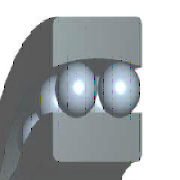
# Autodesk Inventor part: Подшипник 1212 ГОСТ 28428-90
Saved by Autodesk Inventor 2021 (Build 250183000, 183)
## iProperties
Created: 2020-01-21
Part Number: Подшипник 1212 ГОСТ 28428-90
Material: Сталь, мягкая
Description: ПОДШИПНИКИ РАДИАЛЬНЫЕ ШАРИКОВЫЕ СФЕРИЧЕСКИЕ ДВУХРЯДНЫЕ
Document SubType Name: Modeling
Standard: ГОСТ 28428-90
Designer: gdevc
Standards Organization: GOST
Language: ru-RU
Size Designation: 1212
Categories: <MemberInstance><Categories><Category DisplayName="Детали вала" InternalName="7f7aeb1f-a693-4053-b835-cee3144e0d98" Mnemonic="SHFT"><Category DisplayName="Подшипники" InternalName="242d30a3-7172-44e6-a363-b0a3d8f1b556" Mnemonic="BRNG"><CategoryParameter DisplayName="Ширина" InternalName="25fc5f6e-338b-4801-b5ed-8959743e396e" Mnemonic="wdth"/><CategoryParameter DisplayName="Обозначение размера" InternalName="2c4e891a-c8f4-49ed-a5c1-5131476c6feb" Mnemonic="sizedes"/><CategoryParameter DisplayName="Номинальная динамическая нагрузка" InternalName="440972dd-7009-4861-bd45-69ffbb461423" Mnemonic="bdynlrat"/><CategoryParameter DisplayName="Диаметр вала" InternalName="91302473-2833-4451-a660-c5d4a8d6a031" Mnemonic="shaftdia"/><CategoryParameter DisplayName="Угол касания" InternalName="aa21a452-7974-4a55-b5cf-1c2972de2aea" Mnemonic="TouchAngle"/><CategoryParameter DisplayName="Наружный диаметр" InternalName="d441686c-04bd-4681-b674-94fbc173ec23" Mnemonic="outdia"/><Category DisplayName="Подшипники шариковые" InternalName="9b553946-0899-4a5e-a403-c1d9295e77c1" Mnemonic="BALLBEAR"><CategoryParameter DisplayName="Коэффициент радиальной динамической нагрузки при Fa/Fr  &lt;= e" InternalName="051e59b3-bd55-4dad-8b07-38b5cb912881" Mnemonic="raddynfc1"/><CategoryParameter DisplayName="Номинальная статическая нагрузка" InternalName="0f13fbbf-c511-4d43-b4c7-197b47424baf" Mnemonic="bstatlrat"/><CategoryParameter DisplayName="Ресурс" InternalName="3029e2ef-9460-4be8-bdfd-dfe61437473d" Mnemonic="lifeexp"/><CategoryParameter DisplayName="Коэффициент трения" InternalName="3086b0f2-3d69-46ff-8a75-fe12e395bb47" Mnemonic="fricfct"/><CategoryParameter DisplayName="Мин. диаметр вала" InternalName="4a5be9bc-ad86-4bf2-8167-102dad5d3e27" Mnemonic="minshaftdia"/><CategoryParameter DisplayName="Коэффициент осевой динамической нагрузки при Fa/Fr &gt; e" InternalName="4b6ff741-5956-4a40-80f5-34eb9259f88c" Mnemonic="axdynfc2"/><CategoryParameter DisplayName="Ограничивающая скорость смазка" InternalName="5237843b-2c8d-46d3-8227-f3e9dd85a12e" Mnemonic="lubgrsp"/><CategoryParameter DisplayName="Ограничивающее скорость масло" InternalName="60628548-8907-44dc-8e09-603d72f5766f" Mnemonic="oilspd"/><CategoryParameter DisplayName="Коэффициент осевой статической нагрузки" InternalName="74dbf5e2-8362-409a-802f-3c2235668d99" Mnemonic="axdynfc0"/><CategoryParameter DisplayName="Масса" InternalName="7b80f85c-da81-4dea-b8db-d7c689da91b2" Mnemonic="mass"/><CategoryParameter DisplayName="Радиус" InternalName="83352640-dfae-4cba-bc9f-11ecbfb0001c" Mnemonic="rad"/><CategoryParameter DisplayName="Коэффициент радиальной статической нагрузки" InternalName="83ce084d-c51e-4598-a871-e8e1e34b26ee" Mnemonic="raddynfc0"/><CategoryParameter DisplayName="Коэффициент осевой динамической нагрузки при Fa/Fr &lt;= e" InternalName="ae45a7db-08df-4411-99a8-2f035015bff9" Mnemonic="axdynfc1"/><CategoryParameter DisplayName="Макс. диаметр отсека втулки" InternalName="b5cf89e0-ca87-439c-b08c-a25e2999ab06" Mnemonic="maxhubdia"/><CategoryParameter DisplayName="Граничное значение для определения коэффициента" InternalName="be0ce6fc-cad4-4218-b484-c34dd2571812" Mnemonic="limvalfac"/><CategoryParameter DisplayName="Коэффициент радиальной динамической нагрузки при Fa/Fr &gt; e" InternalName="e513bdb7-139f-4b3c-af32-49e0ba1226b9" Mnemonic="raddynfc2"/><CategoryParameter DisplayName="Макс. радиус отсека скругления" InternalName="f6ce6695-cf2c-4ec9-8d20-66671e0e35a4" Mnemonic="maxstprad"/><Category DisplayName="Подшипники шариковые самоустанавливающиеся" InternalName="df14edc0-665f-4502-a2b8-a256b27ec1b7" Mnemonic="BBSABB"/></Category></Category></Category><Category DisplayName="ТипДанных" InternalName="23b78d0f-2648-40c6-8793-ca6db495c9e8" Mnemonic="DATATYPE"><CategoryParameter DisplayName="ОтображаемоеИмя" InternalName="05415f3d-3907-474b-a020-eb9d644f4cf3" Mnemonic="DISPLAYNAME"/><CategoryParameter DisplayName="Стандарт" InternalName="0c0a119c-1e12-4c84-803f-101930972f5e" Mnemonic="STANDARD"/><CategoryParameter DisplayName="Наименование" InternalName="13903e3d-64b1-4950-80da-f627842ea37f" Mnemonic="DESCRIPTION"/><CategoryParameter DisplayName="Обозначение" InternalName="2675968c-4ce5-49e0-a4f5-552d29089031" Mnemonic="DESIGNATION"/><CategoryParameter DisplayName="Строка по умолчанию" InternalName="2af9ec52-faaa-4026-b378-f9fa4afca842" Mnemonic="DEFAULTROW"/><CategoryParameter DisplayName="Имя папки" InternalName="3f06958e-8713-4116-9be7-ed6184ecc97b" Mnemonic="FOLDERNAME"/><CategoryParameter DisplayName="Указатель редакций" InternalName="45a75005-10b1-4dfc-8d6d-dfe629f0b93c" Mnemonic="REVISIONGUID"/><CategoryParameter DisplayName="ИмяФайла" InternalName="8b46a4cc-9585-4fed-90c3-899f57e09a73" Mnemonic="FILENAME"/><CategoryParameter DisplayName="ОргСтанд" InternalName="8f5914e1-4693-403f-8ab5-d37768198c9d" Mnemonic="STDSORG"/><CategoryParameter DisplayName="Версия семейства" InternalName="914462f6-6e19-4b14-ba84-155b9680b1d0" Mnemonic="FAMILYREVISION"/><CategoryParameter DisplayName="Редакция стандарта" InternalName="91d5a463-65c2-4fde-b823-3b7fea5e8e17" Mnemonic="STANDARDREVISION"/><CategoryParameter DisplayName="редакция элемента" InternalName="a65d44b9-392f-4f4f-857b-e4b3d54996fe" Mnemonic="MEMBERREVISION"/><CategoryParameter DisplayName="ФорматКлипа" InternalName="bc51e27b-3422-4e78-93ef-cec197ddf230" Mnemonic="CLIPFORMAT"/><CategoryParameter DisplayName="Изготовитель" InternalName="cd6c7a72-a28a-4e50-99a9-2c7f4e13e5ad" Mnemonic="MANUFACTURER"/><CategoryParameter DisplayName="ВнутреннееИмя" InternalName="cf1d0246-76d9-4b4a-8305-fa0409afb5c1" Mnemonic="INTERNALNAME"/><CategoryParameter DisplayName="Метрическая" InternalName="e2385c5b-1ea4-4823-96a8-8de651266ec3" Mnemonic="ISMETRIC"/><Category DisplayName="Деталь" InternalName="c0e0b642-3bcb-4cc8-9e80-f96d35c4afa4" Mnemonic="PART"><CategoryParameter DisplayName="Номер детали" InternalName="016b6077-bfbe-49bd-92c9-d8d59c39c941" Mnemonic="PARTNUMBER"/><CategoryParameter DisplayName="Инвентарный номер" InternalName="4dba7c1c-e26c-444e-836c-b08b433409a8" Mnemonic="STOCKNUMBER"/><CategoryParameter DisplayName="Ключ материала" InternalName="5c9a8adb-dd2b-4535-b97f-0a94a95fe41f" Mnemonic="MATERIALKEY"/><CategoryParameter DisplayName="Материал" InternalName="818a152a-d3c3-49ca-80ee-df7d91421b8e" Mnemonic="MATERIAL"/></Category></Category></Categories><FamilyTemplate Id="Bearing 1000 GOST 28428-90"><FamilyTemplateParameters><FamilyTemplateParameter ObjectType="kUserParameterObject" ValueType="xs:double" Id="1" ObjectReferenceKey="B"/><FamilyTemplateParameter ObjectType="kUserParameterObject" ValueType="xs:double" Id="2" ObjectReferenceKey="C0"/><FamilyTemplateParameter ObjectType="kUserParameterObject" ValueType="xs:double" Id="3" ObjectReferenceKey="C_"/><FamilyTemplateParameter ObjectType="kUserParameterObject" ValueType="xs:double" Id="4" ObjectReferenceKey="D"/><FamilyTemplateParameter ObjectType="kUserParameterObject" ValueType="xs:double" Id="5" ObjectReferenceKey="d_"/><FamilyTemplateParameter ObjectType="kUserParameterObject" ValueType="xs:double" Id="7" ObjectReferenceKey="r"/><FamilyTemplateParameter ObjectType="kPropertyObject" ValueType="xs:string" Id="100" ObjectReferenceKey="{32853F0F-3444-11d1-9E93-0060B03C1CA6}" SubObjectId="52"/><FamilyTemplateParameter ObjectType="kPropertyObject" ValueType="xs:string" Id="105" ObjectReferenceKey="{32853F0F-3444-11d1-9E93-0060B03C1CA6}" SubObjectId="5"/><FamilyTemplateParameter ObjectType="kPartComponentDefinitionObject" ValueType="xs:string" Id="110" SubObjectId="Material"/></FamilyTemplateParameters></FamilyTemplate><CategoryParameterMap><ParamToTemplateMap><ParamToTemplate CategoryParameter="//CategoryParameter[@InternalName='05415f3d-3907-474b-a020-eb9d644f4cf3']" ConstantValue="Bearing 1000 GOST 28428-90"/><ParamToTemplate CategoryParameter="//CategoryParameter[@InternalName='0c0a119c-1e12-4c84-803f-101930972f5e']" ConstantValue="GOST 28428-90"/><ParamToTemplate CategoryParameter="//CategoryParameter[@InternalName='13903e3d-64b1-4950-80da-f627842ea37f']" ConstantValue="Double-row spherical ball radial bearings"/><ParamToTemplate CategoryParameter="//CategoryParameter[@InternalName='2af9ec52-faaa-4026-b378-f9fa4afca842']" ConstantValue="1"/><ParamToTemplate CategoryParameter="//CategoryParameter[@InternalName='3f06958e-8713-4116-9be7-ed6184ecc97b']" ConstantValue="Bearing 1000 GOST 28428-90"/><ParamToTemplate CategoryParameter="//CategoryParameter[@InternalName='45a75005-10b1-4dfc-8d6d-dfe629f0b93c']" ConstantValue="1b7fd78a-7c81-49d3-bc1e-4460c7399f9d"/><ParamToTemplate CategoryParameter="//CategoryParameter[@InternalName='8f5914e1-4693-403f-8ab5-d37768198c9d']" ConstantValue="GOST"/><ParamToTemplate CategoryParameter="//CategoryParameter[@InternalName='914462f6-6e19-4b14-ba84-155b9680b1d0']" ConstantValue="11"/><ParamToTemplate CategoryParameter="//CategoryParameter[@InternalName='91d5a463-65c2-4fde-b823-3b7fea5e8e17']" TemplateParameter="103"/><ParamToTemplate CategoryParameter="//CategoryParameter[@InternalName='bc51e27b-3422-4e78-93ef-cec197ddf230']" ConstantValue="CF_INVENTOR.STDPARTS"/><ParamToTemplate CategoryParameter="//CategoryParameter[@InternalName='cd6c7a72-a28a-4e50-99a9-2c7f4e13e5ad']" TemplateParameter="104"/><ParamToTemplate CategoryParameter="//CategoryParameter[@InternalName='cf1d0246-76d9-4b4a-8305-fa0409afb5c1']" ConstantValue="0fc8b479-9ddc-4413-bce0-0e3ba5d9839d"/><ParamToTemplate CategoryParameter="//CategoryParameter[@InternalName='e2385c5b-1ea4-4823-96a8-8de651266ec3']" ConstantValue="true"/><ParamToTemplate CategoryParameter="//CategoryParameter[@InternalName='8b46a4cc-9585-4fed-90c3-899f57e09a73']" ConstantValue="Подшипник 1212 ГОСТ 28428-90"/><ParamToTemplate CategoryParameter="//CategoryParameter[@InternalName='a65d44b9-392f-4f4f-857b-e4b3d54996fe']" ConstantValue="eab9ecc3-8d4d-46e1-aeed-24c394f93b6e"/><ParamToTemplate CategoryParameter="//CategoryParameter[@InternalName='25fc5f6e-338b-4801-b5ed-8959743e396e']" TemplateParameter="1"/><ParamToTemplate CategoryParameter="//CategoryParameter[@InternalName='d441686c-04bd-4681-b674-94fbc173ec23']" TemplateParameter="4"/><ParamToTemplate CategoryParameter="//CategoryParameter[@InternalName='2675968c-4ce5-49e0-a4f5-552d29089031']" TemplateParameter="100"/><ParamToTemplate CategoryParameter="//CategoryParameter[@InternalName='2c4e891a-c8f4-49ed-a5c1-5131476c6feb']" TemplateParameter="100"/><ParamToTemplate CategoryParameter="//CategoryParameter[@InternalName='818a152a-d3c3-49ca-80ee-df7d91421b8e']" TemplateParameter="110"/><ParamToTemplate CategoryParameter="//CategoryParameter[@InternalName='016b6077-bfbe-49bd-92c9-d8d59c39c941']" TemplateParameter="105"/><ParamToTemplate CategoryParameter="//CategoryParameter[@InternalName='91302473-2833-4451-a660-c5d4a8d6a031']" TemplateParameter="5"/></ParamToTemplateMap></CategoryParameterMap></MemberInstance>
Mass: 10.0317 g
Surface Area: 18.2999 cm^2
Volume: 1.2763 cm^3
Density: 7.85 g/cm^3
Appearance: С умеренной полировкой
IsCustomPart: 1
Title: Подшипник
Author: gdevc
Autodesk Inventor part; units mm, degrees
ref_plane "YZ Plane" through (0, 0, 0) normal (1, 0, 0) x (0, 1, 0)
ref_plane "XZ Plane" through (0, 0, 0) normal (0, 1, 0) x (-1, 0, 0)
ref_plane "XY Plane" through (0, 0, 0) normal (0, 0, 1) x (1, 0, 0)
sketch "Sketch1" plane through (0, 0, 0) normal (0, 0, 1) x (1, 0, 0)
  line L0 (2.5, 55) -> (19.5, 55)
  line L1 (22, 52.5) -> (22, 45.866)
  line L2 (0, 52.5) -> (0, 45.866)
  line L3 (22, 37.75) -> (22, 32.5)
  line L4 (19.5, 30) -> (2.5, 30)
  line L5 (0, 32.5) -> (0, 37.75)
  arc A0 (22, 45.866) -> (0, 45.866) centre (11, 0) ccw
  line L6 (-5.1249, 0) -> (27.1249, 0) projected
  circle A1 centre (5.5, 42.5208) radius 4.2917
  circle A2 centre (16.5, 42.5208) radius 4.2917
  line L7 (0.8333, 38.5833) -> (3.7927, 38.5833)
  line L8 (7.2073, 38.5833) -> (14.7927, 38.5833)
  line L9 (18.2073, 38.5833) -> (21.1667, 38.5833)
  arc A3 (2.5, 55) -> (0, 52.5) centre (2.5, 52.5) ccw
  arc A4 (22, 52.5) -> (19.5, 55) centre (19.5, 52.5) ccw
  arc A5 (19.5, 30) -> (22, 32.5) centre (19.5, 32.5) ccw
  arc A6 (0, 32.5) -> (2.5, 30) centre (2.5, 32.5) ccw
  line L10 (0.8333, 38.5833) -> (0, 37.75)
  line L11 (21.1667, 38.5833) -> (22, 37.75)
  line L12 (1.2083, 42.5208) -> (9.7917, 42.5208)
  line L13 (12.2083, 42.5208) -> (20.7917, 42.5208)
  line L14 (2.4167, 43.9513) -> (19.5833, 43.9513)
  line L15 (19.5833, 43.9513) -> (19.5833, 41.0902)
  line L16 (19.5833, 41.0902) -> (2.4167, 41.0902)
  line L17 (2.4167, 41.0902) -> (2.4167, 43.9513)
  point P0 (0, 0)
  point P1 (0, 38.5833)
  point P2 (22, 38.5833)
  point P3 (2.4167, 42.5208)
  point P4 (11, 43.9513)
  dimension "d0" = 60
  dimension "d1" = 110
  dimension "d2" = 22
  dimension "d3" = 8.5833
  dimension "d4" = 7.8333
  dimension "d5" = 8.5833
  dimension "d6" = 8.5833
  dimension "d7" = 5.5
  dimension "d8" = 2.5
  dimension "d9" = 0.8333
  dimension "d10" = 0.8333
  dimension "d11" = 0.8333
  dimension "d12" = 0.8333
  dimension "d20" = 2.8611
  dimension "d21" = 17.1667
  constraints: 34 end point, 18 point on circle, 10 tangent, 9 parallel, 8 perpendicular, 7 centre point, 5 collinear, 5 midpoint, 5 point on line, 4 equal radius, 3 horizontal alignment, 2 coincident, 1 horizontal, 1 vertical alignment
  measures "d0" diameter of L4 L6
  measures "d1" diameter of L0 L6
  measures "d2" distance between parallel lines of L1 L2
  measures "d3" distance between parallel lines of L4 L8
  measures "d4" distance edge to line of A0 L0
  measures "d5" distance edge to line of A0 L8
  measures "d6" diameter of A1
  measures "d7" distance from line of L5 A1.centre
  measures "d8" radius of A3
  measures "d9" distance of L7.start point (0, 38.583)
  measures "d10" distance of L5.end point (0, 38.583)
  measures "d11" distance of L9.end point (22, 38.583)
  measures "d12" distance of L3.start point (22, 38.583)
  measures "d20" distance between parallel lines of L16 L14
  measures "d21" distance between parallel lines of L15 L17
revolve "Вращение1" add sketch "Sketch1" angle 360 about axis through (-10, 0, 0) along (1, 0, 0) picked at (4.7932, 43.4745) picked at (17.2068, 43.4745) picked at (4.7932, 41.5671) picked at (17.2068, 41.5671) contours L0 A4 L1 A0 L2 A3 | L14 A2 L16 A1 | A1 L12 L17 L14 | L14 L15 L13 A2 | A1 L16 L17 L12 | A1 L8 A2 L9 L11 L3 A5 L4 A6 L5 L10 L7 | L15 L16 A2 L13
revolve "Вращение2" add sketch "Sketch1" angle 360 about axis through (1.2083, 42.5208, 0) along (1, 0, 0) contours L12 L17 L16 A1 | A2 L16 L15 L13 | A1 L16 L17 L12 | L15 L16 A2 L13
chamfer "Фаска1" distance 1.25 angle 45 2 edges at (0, -45.866, 0) (22, -45.866, 0)
pattern_circular "Круговой Массив1" count 21 over 360 about axis through (11, 0, 0) along (1, 0, 0) of "Вращение2"
equation "\"d0\" = d_"
equation "\"d1\" = D"
equation "\"d2\" = B"
equation "\"d6\" = d5"
equation "\"d7\" = 0.25 * B"
equation "\"d8\" = r"
equation "\"d9\" = 0.333333 * r"
equation "\"d10\" = d9"
equation "\"d11\" = d9"
equation "\"d12\" = d11"
equation "\"d20\" = 0.333333 * d5"
equation "\"d21\" = 2 * d6"
equation "\"d15\" = 0.5 * r"
equation "\"D\" = 110"
equation "\"d_\" = 60"
equation "\"B\" = 22"
equation "\"r\" = 2.5"
body "Solid1"
